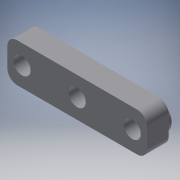
# Autodesk Inventor part: NerfBottomStandoff
Saved by Autodesk Inventor 2018.3 (Build 223284000, 284)
## iProperties
Created: 2019-08-17
Part Number: NerfBottomStandoff
Material: Generic
Document SubType Name: Modeling
Designer: Srinity
Density: 1 g/cm^3
Appearance: Default
Author: Srinity
Autodesk Inventor part; units mm, degrees
ref_plane "YZ Plane" through (0, 0, 0) normal (1, 0, 0) x (0, 1, 0)
ref_plane "XZ Plane" through (0, 0, 0) normal (0, 1, 0) x (-1, 0, 0)
ref_plane "XY Plane" through (0, 0, 0) normal (0, 0, 1) x (1, 0, 0)
sketch "Sketch1" plane through (0, 0, 0) normal (0, 0, 1) x (1, 0, 0)
  circle A0 centre (-40.5918, 0) radius 2.4892 construction
  circle A1 centre (-22.5168, 0) radius 2.4892 construction
  circle A2 centre (-4.4418, 0) radius 2.4892 construction
  circle A3 centre (-40.5918, 0) radius 4.5
  circle A4 centre (-4.4418, 0) radius 4.5
  line L0 (-40.5918, 4.5) -> (-4.4418, 4.5)
  line L1 (-4.4418, 4.5) -> (-4.4418, -4.5)
  line L2 (-4.4418, -4.5) -> (-40.5918, -4.5)
  line L3 (-40.5918, -4.5) -> (-40.5918, 4.5)
  point P0 (0, 0)
  dimension "d1" = 9
  constraints: 8 end point, 3 tangent, 2 centre point, 2 concentric, 2 midpoint, 2 parallel, 1 equal radius, 1 horizontal, 1 perpendicular
  measures "d1" diameter of A3
extrude "Extrusion1" add sketch "Sketch1" along normal blind 1.3
sketch "Sketch2" plane through (0, 0, 1.3) normal (0, 0, 1) x (1, 0, 0)
  line L0 (-45.4068, 6.375) -> (0.3732, 6.375)
  line L1 (0.3732, 6.375) -> (0.3732, -6.375)
  line L2 (0.3732, -6.375) -> (-45.4068, -6.375)
  line L3 (-45.4068, -6.375) -> (-45.4068, 6.375)
  circle A0 centre (-22.5168, 0) radius 2.4892 construction
  point P0 (0, 0)
  dimension "d4" = 45.78
  dimension "d5" = 22.89
  dimension "d6" = 12.75
  dimension "d7" = 6.375
  constraints: 8 end point, 2 parallel, 1 horizontal, 1 perpendicular
  measures "d4" distance of L0.start L0.end
  measures "d5" distance from line of L1 A0.centre
  measures "d6" distance between parallel lines of L2 L0
  measures "d7" distance from line of A0.centre L0
extrude "Extrusion2" add sketch "Sketch2" along normal blind 7.1
fillet "Fillet1" radius 3.175 4 edges at (-45.4068, 6.375, 4.85) (-45.4068, -6.375, 4.85) (0.3732, 6.375, 4.85) (0.3732, -6.375, 4.85)
sketch "Sketch3" plane through (0, 0, 0) normal (0, 0, -1) x (-1, 0, 0)
  circle A0 centre (4.4418, 0) radius 2.4892 construction
  circle A1 centre (22.5168, 0) radius 2.4892 construction
  circle A2 centre (40.5918, 0) radius 2.4892 construction
  circle A3 centre (4.4418, 0) radius 2.794
  circle A4 centre (22.5168, 0) radius 2.794
  circle A5 centre (40.5918, 0) radius 2.794
  point P0 (0, 0)
  dimension "d11" = 5.588
  constraints: 3 centre point, 3 coincident, 2 equal radius
  measures "d11" diameter of A3
extrude "Extrusion3" cut sketch "Sketch3" against normal through all
equation "\"d5\" = 0.5 * d4"
equation "\"d7\" = 0.5 * d6"
body "Solid1"
